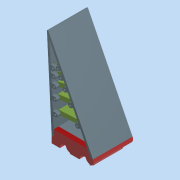
# Autodesk Inventor part: FingerEnclosure
Saved by Autodesk Inventor 2020.3 (Build 243373000, 373)
## iProperties
Created: 2020-03-10
Part Number: FingerEnclosure
Material: Generisch
Document SubType Name: Modeling
Designer: JochenAlt
Density: 1 g/cm^3
Appearance: Rot
Author: JochenAlt
Autodesk Inventor part; units mm, degrees
ref_plane "YZ Plane" through (0, 0, 0) normal (1, 0, 0) x (0, 1, 0)
ref_plane "XZ Plane" through (0, 0, 0) normal (0, 1, 0) x (-1, 0, 0)
ref_plane "XY Plane" through (0, 0, 0) normal (0, 0, 1) x (1, 0, 0)
sketch "MainConstruction" plane through (0, 0, 0) normal (0, 0, 1) x (1, 0, 0)
  line L0 (-44.4573, 0) -> (45.9096, 0) construction
  line L1 (0, -41.3) -> (0, 41.3) construction
  line L2 (-12, 16.3923) -> (12, 16.3923) construction
  line L3 (6, -16.3923) -> (6, -10.3923) construction
  line L4 (6, -10.3923) -> (11.1962, -13.3923) construction
  line L5 (8.1962, -18.5885) -> (11.1962, -13.3923) construction
  line L6 (0, -16.3923) -> (6, -16.3923) construction
  line L7 (-6, -10.3923) -> (-6, -16.3923) construction
  line L8 (-6, -10.3923) -> (-11.1962, -13.3923) construction
  line L9 (0, 16.3923) -> (0, 0) construction
  line L10 (0, 0) -> (0, -16.3923) construction
  line L11 (-12, 14.3923) -> (12, 14.3923) construction
  line L12 (-12, 16.3923) -> (-12, 14.3923) construction
  line L13 (-12, 27) -> (12, 27) construction
  line L14 (-29.3827, -3.1077) -> (-17.3827, -23.8923) construction
  line L15 (0, 16.3923) -> (0, 27) construction
  line L16 (-23.3827, -13.5) -> (-14.1962, -8.1962) construction
  arc A0 (-2.6277, -14.0839) -> (-3.3698, -6.14) centre (-6, -10.3923) ccw construction
  arc A1 (3.3698, -6.14) -> (2.6277, -14.0839) centre (6, -10.3923) ccw construction
  line L17 (-27.2176, -1.8577) -> (-31.5477, -4.3577) construction
  line L18 (-15.2176, -22.6423) -> (-19.5477, -25.1423) construction
  line L19 (19.5477, -25.1423) -> (15.2176, -22.6423) construction
  circle A2 centre (0, 0) radius 22 construction
  line L20 (12, 14.3923) -> (12, 16.3923) construction
  line L21 (23.3827, -13.5) -> (14.1962, -8.1962) construction
  line L22 (20.1962, 2.1962) -> (14.1962, -8.1962) construction
  line L23 (11.1962, -13.3923) -> (14.1962, -8.1962) construction
  line L24 (-6, -16.3923) -> (0, -16.3923) construction
  line L25 (8.1962, -18.5885) -> (15.2176, -22.6423) construction
  line L26 (-15.2176, -22.6423) -> (-8.1962, -18.5885) construction
  line L27 (-12, 29.5) -> (-12, 24.5) construction
  line L28 (12, 29.5) -> (12, 24.5) construction
  line L29 (12, 24.5) -> (12, 16.3923) construction
  line L30 (-12, 24.5) -> (-12, 16.3923) construction
  line L31 (-11.1962, -13.3923) -> (-8.1962, -18.5885) construction
  line L32 (-11.1962, -13.3923) -> (-20.1962, 2.1962) construction
  line L33 (27.2176, -1.8577) -> (31.5477, -4.3577) construction
  line L34 (17.3827, -23.8923) -> (29.3827, -3.1077) construction
  line L35 (27.2176, -1.8577) -> (21.9687, 1.1728) construction
  line L36 (-27.2176, -1.8577) -> (-21.9687, 1.1728) construction
  line L37 (20.1962, 2.1962) -> (21.9687, 1.1728) construction
  line L38 (-21.9687, 1.1728) -> (-20.1962, 2.1962) construction
  line L39 (0, -16.3923) -> (0, -24.5) construction
  line L40 (0, -24.5) -> (0, -29.5) construction
  line L41 (0, -27) -> (24, -27) construction
  line L42 (18.4641, 3.1962) -> (6.4641, -17.5885) construction
  line L43 (-18.4641, 3.1962) -> (-6.4641, -17.5885) construction
  line L44 (-20.1962, 2.1962) -> (-18.4641, 3.1962) construction
  line L45 (20.1962, 2.1962) -> (18.4641, 3.1962) construction
  line L46 (3.3698, -6.14) -> (18.4641, 3.1962) construction
  line L47 (-18.4641, 3.1962) -> (-3.3698, -6.14) construction
  circle A3 centre (30.5, 27) radius 2.5 construction
  line L48 (12, 14.3923) -> (16.25, 14.3923) construction
  line L49 (16.25, 14.3923) -> (31.8962, 24.9262) construction
  line L50 (29.1038, 29.0738) -> (10.2677, 16.3923) construction
  line L51 (12, 16.3923) -> (10.2677, 16.3923) construction
  line L52 (8.1962, -18.5885) -> (6.4641, -17.5885) construction
  line L53 (6.4641, -17.5885) -> (2.6277, -14.0839) construction
  line L54 (-8.1962, -18.5885) -> (-6.4641, -17.5885) construction
  line L55 (-6.4641, -17.5885) -> (-2.6277, -14.0839) construction
  line L56 (4.7294, -16.5869) -> (6.4641, -17.5885) construction
sketch "Main" plane through (0, 0, 0) normal (0, 0, 1) x (1, 0, 0)
  line L0 (-20, 4) -> (-22.8714, 57.5994)
  line L1 (-23, 60) -> (-21.9249, 57.8498) construction
  line L2 (5, 4) -> (-20, 4)
  line L3 (-13.3043, 37.5898) -> (-12.7452, 36.4718)
  line L4 (-19.223, 14.7316) -> (-18.7552, 6)
  line L5 (-19.7847, 25.2166) -> (-19.6509, 22.7202) construction
  line L6 (-19.9933, 29.111) -> (-19.7847, 25.2166)
  line L7 (-6.9724, 24.9261) -> (-3.788, 18.5572)
  line L8 (-10.2496, 31.4804) -> (-8.0904, 27.1622)
  line L9 (-21.3047, 53.5907) -> (-15.7914, 42.5641)
  line L10 (-12.7452, 36.4718) -> (-11.3676, 33.7165)
  line L11 (-21.3047, 53.5907) -> (-20.62, 40.8102)
  line L12 (-20.2672, 34.2237) -> (-20.127, 31.6074)
  line L13 (-3.2289, 17.4392) -> (-2.6699, 16.3212)
  line L14 (-3.788, 18.5572) -> (-3.2289, 17.4392)
  line L15 (-2.6699, 16.3212) -> (2.4907, 6) construction
  line L16 (-19.3567, 17.228) -> (-19.7847, 25.2166) construction
  line L17 (-19.2898, 15.9798) -> (-19.3567, 17.228)
  line L18 (-19.223, 14.7316) -> (-19.2898, 15.9798)
  line L19 (-8.0904, 27.1622) -> (-7.5314, 26.0441)
  line L20 (-7.5314, 26.0441) -> (-6.9724, 24.9261)
  line L21 (-6.9724, 24.9261) -> (-3.788, 18.5572) construction
  line L22 (-19.7847, 25.2166) -> (-19.6509, 22.7202)
  line L23 (-20.127, 31.6074) -> (-20.2672, 34.2237) construction
  line L24 (-20.0602, 30.3592) -> (-20.127, 31.6074)
  line L25 (-19.9933, 29.111) -> (-20.0602, 30.3592)
  line L26 (-11.3676, 33.7165) -> (-10.8086, 32.5985)
  line L27 (-10.8086, 32.5985) -> (-10.2496, 31.4804)
  line L28 (-10.2496, 31.4804) -> (-8.0904, 27.1622) construction
  line L29 (-20.4009, 36.7201) -> (-20.3341, 35.4719)
  line L30 (-13.8633, 38.7079) -> (-13.3043, 37.5898)
  line L31 (-12.7452, 36.4718) -> (-11.3676, 33.7165) construction
  line L32 (-20.2672, 34.2237) -> (-20.3341, 35.4719)
  line L33 (-18.7552, 6) -> (-19.223, 14.7316) construction
  line L34 (-2.6699, 16.3212) -> (2.4907, 6)
  line L35 (-18.7552, 6) -> (2.4907, 6)
  arc A0 (-21.9249, 57.8498) -> (-22.8714, 57.5994) centre (-22.3721, 57.6262) ccw
  line L36 (-18.7552, 6) -> (-18.6481, 4)
  line L37 (2.4907, 6) -> (3.4907, 4)
  circle A1 centre (-12, 0) radius 1.05
  arc A2 (-14.9041, -0.7524) -> (-9, 0) centre (-12, 0) ccw
  circle A3 centre (0, 0) radius 1.05
  arc A4 (-3, 0) -> (3, 0) centre (0, 0) ccw
  line L38 (-9, 0) -> (-3, 0)
  arc A5 (3, 0) -> (5, 4) centre (2.5, 2.75) ccw
  line L39 (-18.7622, 8) -> (1.3789, 8)
  line L40 (-18.6551, 6) -> (-18.7622, 8)
  line L41 (1.3789, 8) -> (2.3789, 6)
  line L42 (-18.6604, 6.1) -> (2.3289, 6.1)
  arc A6 (3, 0) -> (-3, 0) centre (0, 0) ccw
  line L43 (2.1213, 2.1213) -> (3.9075, 0.3352)
  arc A7 (-9, 0) -> (-14.9041, -0.7524) centre (-12, 0) ccw
  line L44 (2.3789, 6) -> (3.3789, 4)
  line L45 (-18.6551, 6) -> (-18.5479, 4)
  line L46 (-20, 4) -> (-20, 0)
  line L47 (-21.9249, 57.8498) -> (5, 4)
  line L48 (-22.8714, 57.5994) -> (-23, 60) construction
  line L49 (-23, 60) -> (-23, 0) construction
  line L50 (0, -47.4) -> (0, 77.9) construction
  line L51 (-44.4573, 0) -> (45.9096, 0) construction
  line L52 (3, 0) -> (-23, 0) construction
  arc A8 (-14.9041, -0.7524) -> (-14.9041, -0.7524) centre (-12, 0) ccw
  line L53 (-15, 0) -> (-20, 0)
  line L54 (-15.2356, 0) -> (-14.7816, 1.1238)
  line L55 (-9.1468, 0.9271) -> (-8.8456, 0)
  line L56 (-8.8456, 0) -> (-9.1468, -0.9271)
  line L57 (-15.2356, 0) -> (-14.7816, -1.1238)
  line L58 (-2.7615, 1.1722) -> (-3.2591, 0)
  line L59 (-2.7615, -1.1722) -> (-3.2591, 0)
  line L60 (-20.4009, 36.7201) -> (-18.9031, 36.8003)
  arc A9 (-18.7693, 34.3039) -> (-18.9031, 36.8003) centre (-18.8362, 35.5521) ccw
  line L61 (-18.7693, 34.3039) -> (-20.2672, 34.2237)
  line L62 (-13.8633, 38.7079) -> (-15.2049, 38.037)
  arc A10 (-15.2049, 38.037) -> (-14.0869, 35.801) centre (-14.6459, 36.919) ccw
  line L63 (-14.0869, 35.801) -> (-12.7452, 36.4718)
  line L64 (-11.3676, 33.7165) -> (-12.7092, 33.0457)
  arc A11 (-12.7092, 33.0457) -> (-11.5912, 30.8096) centre (-12.1502, 31.9276) ccw
  line L65 (-11.5912, 30.8096) -> (-10.2496, 31.4804)
  line L66 (-20.127, 31.6074) -> (-18.6292, 31.6877)
  arc A12 (-18.4954, 29.1912) -> (-18.6292, 31.6877) centre (-18.5623, 30.4395) ccw
  line L67 (-18.4954, 29.1912) -> (-19.9933, 29.111)
  line L68 (-8.0904, 27.1622) -> (-9.4321, 26.4913)
  arc A13 (-9.4321, 26.4913) -> (-8.314, 24.2553) centre (-8.873, 25.3733) ccw
  line L69 (-8.314, 24.2553) -> (-6.9724, 24.9261)
  line L70 (-3.788, 18.5572) -> (-5.1296, 17.8864)
  arc A14 (-5.1296, 17.8864) -> (-4.0116, 15.6503) centre (-4.5706, 16.7684) ccw
  line L71 (-4.0116, 15.6503) -> (-2.6699, 16.3212)
  line L72 (-19.3567, 17.228) -> (-17.8589, 17.3083)
  arc A15 (-17.7251, 14.8119) -> (-17.8589, 17.3083) centre (-17.792, 16.0601) ccw
  line L73 (-17.7251, 14.8119) -> (-19.223, 14.7316)
  circle A16 centre (-14.6459, 36.919) radius 0.5
  circle A17 centre (-18.8362, 35.5521) radius 0.5
  circle A18 centre (-18.5623, 30.4395) radius 0.5
  circle A19 centre (-12.1502, 31.9276) radius 0.5
  circle A20 centre (-8.873, 25.3733) radius 0.5
  circle A21 centre (-17.792, 16.0601) radius 0.5
  circle A22 centre (-4.5706, 16.7684) radius 0.5
  line L74 (-18.8362, 35.5521) -> (-14.6459, 36.919) construction
  line L75 (-18.5623, 30.4395) -> (-12.1502, 31.9276) construction
  line L76 (-17.792, 16.0601) -> (-4.5706, 16.7684) construction
  circle A23 centre (-19.305, 39.6289) radius 0.5
  line L77 (-19.3718, 40.8771) -> (-20.62, 40.8102)
  line L78 (-20.4863, 38.3138) -> (-19.2381, 38.3807)
  arc A24 (-19.2381, 38.3807) -> (-19.3718, 40.8771) centre (-19.305, 39.6289) ccw
  line L79 (-20.4863, 38.3138) -> (-20.4009, 36.7201)
  line L80 (-20.62, 40.8102) -> (-20.4863, 38.3138)
  circle A25 centre (-16.3504, 40.8871) radius 0.5
  arc A26 (-16.9094, 42.0051) -> (-15.7914, 39.769) centre (-16.3504, 40.8871) ccw
  line L81 (-16.9094, 42.0051) -> (-15.7914, 42.5641)
  line L82 (-15.7914, 39.769) -> (-14.6734, 40.328)
  line L83 (-14.6734, 40.328) -> (-13.8633, 38.7079)
  line L84 (-15.7914, 42.5641) -> (-14.6734, 40.328)
  line L85 (-19.305, 39.6289) -> (-16.3504, 40.8871) construction
  circle A27 centre (-18.2199, 24.0486) radius 0.5
  line L86 (-18.2868, 25.2968) -> (-19.7847, 25.2166)
  line L87 (-18.1531, 22.8004) -> (-19.6509, 22.7202)
  line L88 (-19.6509, 22.7202) -> (-19.3567, 17.228)
  line L89 (-18.2199, 24.0486) -> (-8.873, 25.3733) construction
  line L90 (-18.7622, 8) -> (-18.8621, 7.9947)
  line L91 (1.3789, 8) -> (1.4907, 8)
  line L92 (-19.7847, 25.2166) -> (-19.6509, 22.7202)
  line L93 (-18.2199, 24.0486) -> (-19.7178, 23.9684) construction
  line L94 (-18.5623, 30.4395) -> (-20.2321, 30.35) construction
  line L95 (-18.8362, 35.5521) -> (-20.3341, 35.4719) construction
  line L96 (-19.305, 39.6289) -> (-20.5532, 39.562) construction
  line L97 (-19.2898, 15.9798) -> (-17.792, 16.0601) construction
  arc A28 (-18.1531, 22.8004) -> (-18.2868, 25.2968) centre (-18.2199, 24.0486) ccw
  point P0 (-20.0171, 4.3184)
  point P1 (-18.5329, 1.8501)
  point P2 (0, 3)
  point P3 (-12, 3)
  point P4 (3.5032, 0.0324)
  point P5 (-16.5, 4)
  point P6 (-8.8456, 0)
  point P7 (-3.2591, 0)
  point P8 (-3.2591, 0)
  point P9 (-14.9041, -0.7524)
  point P10 (-18.8621, 7.9947)
  point P11 (2.9997, 0.0406)
  point P12 (-19.5609, 21.0395)
  dimension "d29" = 1.35
  dimension "d30" = 1.35
  dimension "d45" = 0.5
  dimension "d46" = 2
  dimension "d112" = 2.1
  dimension "d114" = 12
  dimension "d124" = 2
  dimension "d127" = 0.1
  dimension "d128" = 0.1
  dimension "d129" = 0.1
  dimension "d133" = 25
  dimension "d138" = 60
  dimension "d141" = 10
  dimension "d144" = 5.12
  dimension "d145" = 8
  dimension "d147" = 68
  dimension "d148" = 135
  dimension "d149" = 72
  dimension "d150" = 67
  dimension "d151" = 3
  dimension "d152" = 4
  dimension "d154" = 3
  dimension "d155" = 1
  dimension "d156" = 1.25
  dimension "d164" = 70
  dimension "d165" = 5
  dimension "d166" = 5
  dimension "d167" = 5
  dimension "d168" = 5
  dimension "d176" = 8
  dimension "d177" = 6.4
  dimension "d178" = 4.096
  dimension "d179" = 1.5
  constraints: 194 end point, 166 collinear, 45 point on circle, 41 tangent, 33 perpendicular, 31 point on line, 29 centre point, 22 equal radius, 21 coincident, 15 equal length, 6 horizontal, 6 parallel, 2 midpoint, 1 vertical, 9 other
  measures "d29" distance between parallel lines of L0 L11
  measures "d30" distance between parallel lines of L1 L9
  measures "d45" radius of A0
  measures "d46" distance between parallel lines of L2 L35
  measures "d112" diameter of A1
  measures "d114" distance of A3.centre A1.centre
  measures "d124" distance between parallel lines of L39 L35
  measures "d127" distance between parallel lines of L40 L4
  measures "d128" distance between parallel lines of L34 L41
  measures "d129" distance between parallel lines of L42 L35
  measures "d133" distance of L2.start L0.start
  measures "d138" distance of L1.start L49.end
  measures "d141" distance of L17.start L40.start
  measures "d144" distance of L32.end L24.start
  measures "d145" distance from line of A7.centre L46
  measures "d147" angle of L53 L54
  measures "d148" angle of L51 L43
  measures "d149" angle of L38 L55
  measures "d150" angle of L38 L58
  measures "d151" radius of A2
  measures "d152" distance between parallel lines of L2 L52
  measures "d154" distance of L46.end L49.end
  measures "d155" diameter of A16
  measures "d156" radius of A10
  measures "d164" angle of L85 L11
  measures "d165" angle of L89 L75
  measures "d166" angle of L76 L89
  measures "d167" angle of L74 L85
  measures "d168" angle of L75 L74
  measures "d176" distance of L17.start L93.end
  measures "d177" distance of L93.end L24.start
  measures "d178" distance of L32.end L96.end
  measures "d179" distance of L29.start L60.end
extrude "Extrusion1" add sketch "Main" along normal mid plane 18 contours L0 A0 L47 L2 L37 L34 L13 L14 L7 L20 L19 L8 L27 L26 L10 L3 L30 L83 L84 L9 L11 L80 L79 L29 L32 L12 L24 L25 L6 L22 L88 L17 L18 L4 L36 | L36 L35 L45 L2 | L45 L35 L44 L2 | L4 L90 L40 L35 | L44 L35 L37 L2 | L40 L42 L41 L35 | L41 L91 L34 L35 | L40 L39 L41 L42 | L18 L17 L72 A15 L73 | L71 A14 L70 L14 L13 | L22 L86 A28 L87 | L25 L24 L66 A12 L67 | L69 A13 L68 L19 L20 | L32 L29 L60 A9 L61 | L65 A11 L64 L26 L27 | L80 L77 A24 L78 | L63 A10 L62 L30 L3 | L84 L82 A26 L81
extrude "Extrusion16" add sketch "Main" along normal mid plane 24 contours L0 A0 L47 L2 L37 L34 L13 L14 L7 L20 L19 L8 L27 L26 L10 L3 L30 L83 L84 L9 L11 L80 L79 L29 L32 L12 L24 L25 L6 L22 L88 L17 L18 L4 L36 | L18 L17 L72 A15 L73 | L71 A14 L70 L14 L13 | L22 L86 A28 L87 | L25 L24 L66 A12 L67 | L69 A13 L68 L19 L20 | L32 L29 L60 A9 L61 | L65 A11 L64 L26 L27 | L80 L77 A24 L78 | L63 A10 L62 L30 L3 | L84 L82 A26 L81
extrude "Extrusion22" cut sketch "Main" against normal mid plane 20 contours L18 L17 L72 A15 L73 | L71 A14 L70 L14 L13 | L22 L86 A28 L87 | L25 L24 L66 A12 L67 | L69 A13 L68 L19 L20 | L32 L29 L60 A9 L61 | L65 A11 L64 L26 L27 | L80 L77 A24 L78 | L63 A10 L62 L30 L3 | L84 L82 A26 L81
extrude "Extrusion17" add sketch "Main" along normal mid plane 17 separate body contours L2 A5 L43 A6 L58 L38 L55 A7 L54 L53 L46 | L54 A7 L53 | A7 A2 | A5 A6 L43 | L55 L38 A7 | A2 L38 L56 | A4 A6 | L59 L38 A4 | A6 L38 L58
extrude "Extrusion18" add sketch "Main" along normal mid plane 24 contours L2 A5 L43 A6 L58 L38 L55 A7 L54 L53 L46 | L45 L35 L44 L2 | L54 A7 L53 | L40 L42 L41 L35 | A5 A6 L43 | L40 L39 L41 L42 bodies 2
extrude "Extrusion19" cut sketch "Main" along normal mid plane 20.25 contours L36 L35 L45 L2 | L45 L35 L44 L2 | L44 L35 L37 L2 | L40 L42 L41 L35 bodies 2
extrude "Extrusion20" cut sketch "Main" along normal mid plane 18 contours L40 L42 L41 L35 | L40 L39 L41 L42 bodies 2
sketch "rig" plane through (0, 0, 0) normal (0, 0, 1) x (1, 0, 0)
  circle A0 centre (-18.8362, 35.5521) radius 0.5 projected
  circle A1 centre (-19.305, 39.6289) radius 0.5 projected
  circle A2 centre (-16.3504, 40.8871) radius 0.5 projected
  circle A3 centre (-14.6459, 36.919) radius 0.5 projected
  circle A4 centre (-12.1502, 31.9276) radius 0.5 projected
  circle A5 centre (-8.873, 25.3733) radius 0.5 projected
  circle A6 centre (-18.2199, 24.0486) radius 0.5 projected
  circle A7 centre (-17.792, 16.0601) radius 0.5 projected
  circle A8 centre (-4.5706, 16.7684) radius 0.5 projected
  line L0 (-17.8589, 17.3083) -> (-4.6374, 18.0166)
  arc A9 (-4.5037, 15.5202) -> (-4.6374, 18.0166) centre (-4.5706, 16.7684) ccw
  line L1 (-4.5037, 15.5202) -> (-17.7251, 14.8119)
  arc A10 (-17.8589, 17.3083) -> (-17.7251, 14.8119) centre (-17.792, 16.0601) ccw
  line L2 (-18.3953, 25.2863) -> (-9.0485, 26.6109)
  line L3 (-18.0445, 22.811) -> (-8.6976, 24.1357)
  arc A11 (-18.3953, 25.2863) -> (-18.0445, 22.811) centre (-18.2199, 24.0486) ccw
  arc A12 (-8.6976, 24.1357) -> (-9.0485, 26.6109) centre (-8.873, 25.3733) ccw
  line L4 (-18.8449, 31.6571) -> (-12.4328, 33.1453)
  line L5 (-18.2797, 29.2218) -> (-11.8676, 30.71)
  arc A13 (-18.8449, 31.6571) -> (-18.2797, 29.2218) centre (-18.5623, 30.4395) ccw
  arc A14 (-11.8676, 30.71) -> (-12.4328, 33.1453) centre (-12.1502, 31.9276) ccw
  circle A15 centre (-18.5623, 30.4395) radius 0.5 projected
  line L6 (-18.4486, 34.3638) -> (-14.2583, 35.7306)
  arc A16 (-14.2583, 35.7306) -> (-15.0336, 38.1074) centre (-14.6459, 36.919) ccw
  line L7 (-15.0336, 38.1074) -> (-19.2239, 36.7405)
  arc A17 (-19.2239, 36.7405) -> (-18.4486, 34.3638) centre (-18.8362, 35.5521) ccw
  arc A18 (-19.7947, 40.7789) -> (-18.8152, 38.4788) centre (-19.305, 39.6289) ccw
  arc A19 (-15.8607, 39.737) -> (-16.8402, 42.0371) centre (-16.3504, 40.8871) ccw
  line L8 (-19.7947, 40.7789) -> (-16.8402, 42.0371)
  line L9 (-18.8152, 38.4788) -> (-15.8607, 39.737)
  point P0 (0, 0)
  dimension "d173" = 2.5
  constraints: 21 end point, 20 point on circle, 20 tangent, 10 centre point, 10 coincident, 5 equal radius, 4 parallel
  measures "d173" distance between parallel lines of L1 L0
extrude "Extrusion23" add sketch "rig" along normal mid plane 19 separate body
equation "\"d30\" = d29"
equation "\"d5\" = d20"
equation "\"roundness_small\" = 3"
equation "\"roundness_tiny\" = 0.5"
equation "\"wall_thickness\" = 3"
equation "\"medium_arm_width\" = 51"
equation "\"big_arm_width\" = 56"
equation "\"bevel_angle\" = 20deg"
equation "\"medium_arm_radius\" = 35"
equation "\"big_arm_radius\" = 48"
equation "\"medium_arm_circle_centre\" = 11"
equation "\"big_arm_circle_centre\" = 25"
equation "\"thickness\" = 3"
equation "\"tight_fit\" = 0.2"
equation "\"press_fit\" = 0.1"
equation "\"m2_screw_hole_diameter\" = 2.2"
equation "\"m2_hex_width\" = 4.2"
equation "\"m2_washer_diameter\" = 5.2"
equation "\"m2_allen_screw_width\" = 4"
equation "\"m2_allen_screw_height\" = 2"
equation "\"m2_washer_height\" = 0.3"
equation "\"d20\" = 1"
